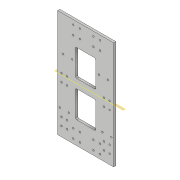
# Autodesk Inventor part: Gripper Back
Saved by Autodesk Inventor 2018 (Build 220112000, 112)
## iProperties
Created: 2017-12-20
Part Number: Gripper Back
Material: Generic
Document SubType Name: Modeling
Designer: dsayers
Density: 1 g/cm^3
Appearance: Default
Author: dsayers
Autodesk Inventor part; units mm, degrees
ref_plane "YZ Plane" through (0, 0, 0) normal (1, 0, 0) x (0, 1, 0)
ref_plane "XZ Plane" through (0, 0, 0) normal (0, 1, 0) x (-1, 0, 0)
ref_plane "XY Plane" through (0, 0, 0) normal (0, 0, 1) x (1, 0, 0)
sketch "Sketch1" plane through (0, 0, 0) normal (0, 0, 1) x (1, 0, 0)
  line L0 (0, 0) -> (158.75, 0)
  line L1 (158.75, 0) -> (158.75, 304.8)
  line L2 (158.75, 304.8) -> (0, 304.8)
  line L3 (0, 304.8) -> (0, 0)
  dimension "d0" = 158.75
  dimension "d1" = 304.8
  constraints: 8 end point, 2 parallel, 1 horizontal, 1 perpendicular
  measures "d0" distance of L1.end L2.end
  measures "d1" distance of L0.end L1.end
extrude "Extrusion1" add sketch "Sketch1" along normal blind 6.35
sketch "Sketch2" plane through (0, 0, 0) normal (0, 0, -1) x (-1, 0, 0)
  circle A0 centre (-117.475, 205.8824) radius 2.4638 projected
  line L0 (-177.2766, 228.1074) -> (-172.9586, 228.1074) projected
  circle A1 centre (-142.875, 205.8824) radius 2.4638 projected
  circle A2 centre (-41.275, 205.8824) radius 2.4638 projected
  circle A3 centre (-15.875, 205.8824) radius 2.4638 projected
  circle A4 centre (-147.6375, 26.9875) radius 2.4638 projected
  circle A5 centre (-131.7625, 26.9875) radius 2.4638 projected
  circle A6 centre (-131.7625, 49.2125) radius 2.4638 projected
  circle A7 centre (-147.6375, 49.2125) radius 2.4638 projected
  circle A8 centre (-26.9875, 26.9875) radius 2.4638 projected
  circle A9 centre (-11.1125, 26.9875) radius 2.4638 projected
  circle A10 centre (-11.1125, 49.2125) radius 2.4638 projected
  circle A11 centre (-26.9875, 49.2125) radius 2.4638 projected
  circle A12 centre (-11.1125, 156.6699) radius 2.4638 projected
  circle A13 centre (-11.1125, 134.4449) radius 2.4638 projected
  circle A14 centre (-26.9875, 134.4449) radius 2.4638 projected
  circle A15 centre (-26.9875, 156.6699) radius 2.4638 projected
  circle A16 centre (-147.6375, 134.4449) radius 2.4638 projected
  circle A17 centre (-131.7625, 134.4449) radius 2.4638 projected
  circle A18 centre (-147.6375, 156.6699) radius 2.4638 projected
  circle A19 centre (-131.7625, 156.6699) radius 2.4638 projected
  point P0 (0, 0)
sketch "Sketch3" plane through (0, 0, 0) normal (0, 0, -1) x (-1, 0, 0)
  line L0 (47.625, 49.2116) -> (-206.375, 49.2116) projected
  point P0 (0, 0)
  point P1 (-142.875, 205.8824)
  point P2 (-117.475, 205.8824)
  point P3 (-131.7625, 156.6699)
  point P4 (-147.6375, 156.6699)
  point P5 (-147.6375, 134.4449)
  point P6 (-131.7625, 134.4449)
  point P7 (-147.6375, 49.2125)
  point P8 (-131.7625, 49.2125)
  point P9 (-131.7625, 26.9875)
  point P10 (-147.6375, 26.9875)
  point P11 (-26.9875, 26.9875)
  point P12 (-11.1125, 26.9875)
  point P13 (-11.1125, 49.2125)
  point P14 (-26.9875, 49.2125)
  point P15 (-26.9875, 134.4449)
  point P16 (-11.1125, 134.4449)
  point P17 (-11.1125, 156.6699)
  point P18 (-26.9875, 156.6699)
  point P19 (-41.275, 205.8824)
  point P20 (-15.875, 205.8824)
hole "Hole1" at (142.875, 205.8824, 0) at (117.475, 205.8824, 0) at (41.275, 205.8824, 0) at (15.875, 205.8824, 0) at (26.9875, 156.6699, 0) at (11.1125, 156.6699, 0) at (11.1125, 134.4449, 0) at (26.9875, 134.4449, 0) at (131.7625, 156.6699, 0) at (147.6375, 156.6699, 0) at (131.7625, 134.4449, 0) at (147.6375, 134.4449, 0) at (147.6375, 49.2125, 0) at (131.7625, 49.2125, 0) at (131.7625, 26.9875, 0) at (147.6375, 26.9875, 0) at (26.9875, 26.9875, 0) at (11.1125, 26.9875, 0) at (11.1125, 49.2125, 0) at (26.9875, 49.2125, 0) direction (0, 0, 1) diameter 4.4958 depth 25.4 tip angle 118 clearance for "Flat Head Machine Screw (82)" size "#8" standard "Ansi Unified Screw Threads"
sketch "Sketch4" plane through (0, 0, 0) normal (0, 0, -1) x (-1, 0, 0)
  circle A0 centre (-11.1125, 49.2125) radius 2.2479 projected
  circle A1 centre (-26.9875, 26.9875) radius 2.2479 projected
  circle A2 centre (-131.7625, 26.9875) radius 2.2479 projected
  circle A3 centre (-147.6375, 49.2125) radius 2.2479 projected
  circle A4 centre (-131.7625, 134.4449) radius 2.2479 projected
  circle A5 centre (-131.7625, 156.6699) radius 2.2479 projected
  circle A6 centre (-11.1125, 134.4449) radius 2.2479 projected
  circle A7 centre (-26.9875, 156.6699) radius 2.2479 projected
  circle A8 centre (-41.275, 205.8824) radius 2.2479 projected
  circle A9 centre (-142.875, 205.8824) radius 2.2479 projected
  circle A10 centre (-117.475, 205.8824) radius 2.2479 projected
  circle A11 centre (-15.875, 205.8824) radius 2.2479 projected
  circle A12 centre (-11.1125, 156.6699) radius 2.2479 projected
  circle A13 centre (-26.9875, 134.4449) radius 2.2479 projected
  circle A14 centre (-147.6375, 156.6699) radius 2.2479 projected
  circle A15 centre (-147.6375, 134.4449) radius 2.2479 projected
  circle A16 centre (-131.7625, 49.2125) radius 2.2479 projected
  circle A17 centre (-147.6375, 26.9875) radius 2.2479 projected
  circle A18 centre (-11.1125, 26.9875) radius 2.2479 projected
  circle A19 centre (-26.9875, 49.2125) radius 2.2479 projected
  line L0 (0, 0) -> (-158.75, 0) projected
  line L1 (0, 304.8) -> (0, 0) projected
  line L2 (-158.75, 304.8) -> (0, 304.8) projected
  line L3 (-158.75, 0) -> (-158.75, 304.8) projected
  line L4 (-82.55, 718.8359) -> (-82.55, -134.6309)
  line L5 (0, 0) -> (-158.75, 0) projected
  point P0 (-120.65, 38.1)
  point P1 (-120.65, 12.7)
  point P2 (-44.45, 38.1)
  point P3 (-44.45, 12.7)
  point P4 (-101.6, 38.1)
  point P5 (-63.5, 38.1)
  point P6 (-63.5, 12.7)
  point P7 (-101.6, 12.7)
  dimension "d11" = 19.05
  dimension "d12" = 19.05
  dimension "d13" = 19.05
  dimension "d14" = 19.05
  dimension "d15" = 19.05
  dimension "d16" = 19.05
  dimension "d17" = 19.05
  dimension "d18" = 19.05
  dimension "d19" = 25.4
  dimension "d20" = 25.4
  dimension "d21" = 12.7
  dimension "d22" = 12.7
  dimension "d23" = 12.7
  dimension "d24" = 12.7
  constraints: 2 end point, 1 vertical, 2 other
  measures "d11" distance of point (-120.65, 38.1) point (-101.6, 38.1)
  measures "d12" distance from line of point (-101.6, 38.1) L4
  measures "d13" distance from line of L4 point (-63.5, 38.1)
  measures "d14" distance of point (-63.5, 38.1) point (-44.45, 38.1)
  measures "d15" distance of point (-63.5, 12.7) point (-44.45, 12.7)
  measures "d16" distance from line of L4 point (-63.5, 12.7)
  measures "d17" distance from line of L4 point (-101.6, 12.7)
  measures "d18" distance of point (-120.65, 12.7) point (-101.6, 12.7)
  measures "d19" distance of point (-101.6, 12.7) point (-101.6, 38.1)
  measures "d20" distance of point (-63.5, 38.1) point (-63.5, 12.7)
  measures "d21" distance from line of L0 point (-101.6, 12.7)
  measures "d22" distance from line of L0 point (-63.5, 12.7)
  measures "d23" distance from line of L0 point (-44.45, 12.7)
  measures "d24" distance from line of L5 point (-120.65, 12.7)
hole "Hole2" at (120.65, 38.1, 0) at (120.65, 12.7, 0) at (44.45, 38.1, 0) at (44.45, 12.7, 0) at (101.6, 38.1, 0) at (63.5, 38.1, 0) at (63.5, 12.7, 0) at (101.6, 12.7, 0) direction (0, 0, 1) diameter 4.4958 depth 25.4 tip angle 118 clearance for "Flat Head Machine Screw (82)" size "#8" standard "Ansi Unified Screw Threads"
ref_plane "Work Plane1" through (0, 152.4, 0) normal (0, 1, 0) x (1, 0, 0)
mirror "Mirror1" about plane through (0, 152.4, 0) normal (0, 1, 0) of "Hole2"
sketch "Sketch5" plane through (0, 0, 0) normal (0, 0, -1) x (-1, 0, 0)
  line L0 (-107.95, 241.3) -> (-50.8, 241.3)
  line L1 (-50.8, 241.3) -> (-50.8, 63.5)
  line L2 (-50.8, 63.5) -> (-107.95, 63.5)
  line L3 (-107.95, 63.5) -> (-107.95, 241.3)
  line L4 (0, 0) -> (-158.75, 0) projected
  line L5 (-158.75, 304.8) -> (0, 304.8) projected
  line L6 (0, 304.8) -> (0, 0) projected
  line L7 (-158.75, 0) -> (-158.75, 304.8) projected
  dimension "d32" = 63.5
  dimension "d33" = 63.5
  dimension "d34" = 50.8
  dimension "d35" = 50.8
  constraints: 8 end point, 2 parallel, 1 horizontal, 1 perpendicular
  measures "d32" distance between parallel lines of L4 L2
  measures "d33" distance between parallel lines of L5 L0
  measures "d34" distance between parallel lines of L6 L1
  measures "d35" distance between parallel lines of L7 L3
extrude "Extrusion2" cut sketch "Sketch5" against normal blind 6.35 contours L0 L1 L2 L3
sketch "Sketch6" plane through (0, 0, 0) normal (0, 0, -1) x (-1, 0, 0)
  line L0 (-107.95, 63.5) -> (-107.95, 241.3) projected
  line L1 (-50.8, 241.3) -> (-50.8, 63.5) projected
  line L2 (-107.95, 165.1) -> (-50.8, 165.1)
  line L3 (-50.8, 165.1) -> (-50.8, 139.7)
  line L4 (-50.8, 139.7) -> (-107.95, 139.7)
  line L5 (-107.95, 139.7) -> (-107.95, 165.1)
  line L6 (-212.7319, 152.4) -> (35.4553, 152.4) projected
  point P0 (0, 0)
  dimension "d38" = 12.7
  dimension "d39" = 12.7
  constraints: 8 end point, 2 parallel, 2 point on line, 1 horizontal, 1 perpendicular
  measures "d38" distance between parallel lines of L6 L2
  measures "d39" distance between parallel lines of L6 L4
extrude "Extrusion3" add sketch "Sketch6" against normal up to surface (6.35 mm away)
fillet "Fillet1" radius 3.175 4 edges at (50.8, 241.3, 3.175) (107.95, 241.3, 3.175) (107.95, 165.1, 3.175) (50.8, 165.1, 3.175)
fillet "Fillet2" radius 3.175 4 edges at (107.95, 139.7, 3.175) (50.8, 139.7, 3.175) (107.95, 63.5, 3.175) (50.8, 63.5, 3.175)
sketch "Sketch7" plane through (0, 0, 0) normal (0, 0, -1) x (-1, 0, 0)
  line L0 (0, 0) -> (-158.75, 0) projected
  line L1 (0, 304.8) -> (0, 0) projected
  line L2 (-158.75, 0) -> (-158.75, 304.8) projected
  point P0 (-127, 69.85)
  point P1 (-152.4, 69.85)
  point P2 (-6.35, 69.85)
  point P3 (-31.75, 69.85)
  dimension "d44" = 25.4
  dimension "d45" = 69.85
  dimension "d46" = 69.85
  dimension "d47" = 69.85
  dimension "d48" = 69.85
  dimension "d49" = 25.4
  dimension "d50" = 6.35
  dimension "d51" = 6.35
  measures "d44" distance of point (-127, 69.85) point (-152.4, 69.85)
  measures "d45" distance from line of L0 point (-152.4, 69.85)
  measures "d46" distance from line of L0 point (-127, 69.85)
  measures "d47" distance from line of L0 point (-6.35, 69.85)
  measures "d48" distance from line of L0 point (-31.75, 69.85)
  measures "d49" distance of point (-31.75, 69.85) point (-6.35, 69.85)
  measures "d50" distance from line of L1 point (-6.35, 69.85)
  measures "d51" distance from line of L2 point (-152.4, 69.85)
hole "Hole3" at (127, 69.85, 0) at (152.4, 69.85, 0) at (6.35, 69.85, 0) at (31.75, 69.85, 0) direction (0, 0, 1) diameter 4.4958 depth 25.4 tip angle 118 clearance for "Flat Head Machine Screw (82)" size "#8" standard "Ansi Unified Screw Threads"
equation "\"d14\" = d11"
equation "\"d15\" = d14"
equation "\"d16\" = d14"
equation "\"d17\" = d11"
equation "\"d18\" = d11"
equation "\"d20\" = d19"
equation "\"d22\" = d21"
equation "\"d23\" = d22"
equation "\"d24\" = d21"
equation "\"d39\" = d38"
equation "\"d46\" = d45"
equation "\"d47\" = d46"
equation "\"d48\" = d47"
equation "\"d49\" = d44"
body "Solid1"
